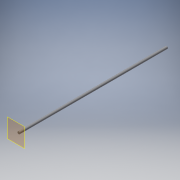
# Autodesk Inventor part: Spinner Rail
Saved by Autodesk Inventor 2016 (Build 200138000, 138)
## iProperties
Created: 2016-07-16
Part Number: Spinner Rail
Material: Generic
Document SubType Name: Modeling
Designer: Scott
Density: 1 g/cm^3
Appearance: Default
Author: Scott
Autodesk Inventor part; units mm, degrees
ref_plane "YZ Plane" through (0, 0, 0) normal (1, 0, 0) x (0, 1, 0)
ref_plane "XZ Plane" through (0, 0, 0) normal (0, 1, 0) x (-1, 0, 0)
ref_plane "Work Plane1" through (0, 0, 0) normal (0, 0, 1) x (1, 0, 0)
sketch "Sketch1" plane through (0, 0, 0) normal (0, 0, 1) x (1, 0, 0)
  circle A0 centre (10.89, 0) radius 11 projected
  line L0 (26.765, 10.283) -> (14.065, 22.983) projected
  line L1 (-22.0025, 22.983) -> (14.065, 22.983) projected
  line L2 (-22.0025, 22.983) -> (-22.0025, -30.992) projected
  line L3 (26.765, -30.992) -> (-22.0025, -30.992) projected
  line L4 (26.765, 10.283) -> (26.765, -30.992) projected
  circle A1 centre (10.89, 0) radius 4
  point P0 (0, 0)
  dimension "d0" = 8
  constraints: 1 centre point, 1 coincident
  measures "d0" diameter of A1
ref_plane "Work Plane2" through (-22.0025, -30.992, -465.865) normal (0, 0, -1) x (0, 1, 0)
extrude "Extrusion1" add sketch "Sketch1" against normal up to surface (465.865 mm away) contours A1
body "Solid1"
